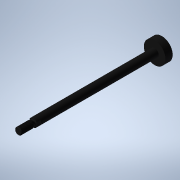
# Autodesk Inventor part: 1463250 DSBC-32-100_(K)
Saved by Autodesk Inventor 2021 (Build 250183000, 183)
## iProperties
Created: 2025-06-06
Part Number: 1463250 DSBC-32-100_(K)
Material: Generic
Catalog Web Link: www.cadenas.de
Description: DSBC_K-Standard cylinder
Vendor: FESTO
Document SubType Name: Modeling
Designer: psAdmin
Manufacturer: FESTO
Mass: 30.5799 g
Surface Area: 101.586 cm^2
Volume: 30.5799 cm^3
Density: 1 g/cm^3
Appearance: PSOLRGB-128-128-128
Category: PARTsolutions
Company: FESTO
Title: 1463250 DSBC-32-100_(K)
Author: Cadenas PARTsolutions
Comments: Standard cylinder
PSOL_IDENT_0: {$CADENAS_DATA/23d-libs/festo/parts/d/dsbc/parts/dsbc_kst.prj},223 {VTYP=3D},{NB=1463250 DSBC-32-100
PSOL_IDENT_1: _(K)},{LINA=1463250 DSBC-32-100_(K)},{NN=DSBC_K},{DATE=30.04.2025 10:56:01},{GEOMDATE=14.10.2015 11:
PSOL_IDENT_2: 10:00},{VERSION=},{LINEID=10},{WBVAR=HUB,VER,FES,KA,KGA,PAR,EG,EK},{WBNUMERIC=HUB,EG,EK}  {NB=146325
PSOL_IDENT_3: 0 DSBC-32-100_(K)},{LINA=1463250 DSBC-32-100_(K)},{KT=DUMMY},{TNR=1463250},{TYP=DSBC},{KDM=32},{HUB=
PSOL_IDENT_4: 100},{HUBMIN=1},{HUBMAX=2800},{VER=-},{VERT=},{FES=-},{FEST=},{KA=-},{KAT=},{KGA=-},{KGAT=},{PAR=-},
PSOL_IDENT_5: {PAR1='-','P2'},{PART=},{EG=0},{EGT=},{A1=35},{EK=0},{EKT=},{A2=0},{A2N=500},{A2P=0},{A=22},{AM=22},
PSOL_IDENT_6: {AF=12},{B=30},{BG=16},{E=45},{EE=G1/8},{EEK=9.728},{G=28.0},{H1=5},{KK=M10x1.25},{KKDM=10.000},{KKP=
PSOL_IDENT_7: 1.250},{L2=18.0},{L3=4.0},{L7=6.5},{L8N=94.000},{L8=194.000},{MM=12},{PL=19.5},{RT=M6},{RTK=6.000},{
PSOL_IDENT_8: TG=32.5},{VA=4},{VD=10.0},{WH=26.0},{ZJN=119.100},{ZJ=219.100},{ZMN=146.100},{ZM=346.100},{SW1=10},{
PSOL_IDENT_9: SW2=16},{SW3=6},{D1=6.4},{KF=M6},{KFK=6.000},{T1=16.0},{T2=2.6},{WL=6.000},{C3=8.200},{D5=1.500},{E2=
PSOL_IDENT_10: 20.000},{F2=0.600},{QH=10.000},{QR=1.000},{W3=45.000},{FDTPIRODACC=4.000},{FDTBDIN439=5.000}
NB: 1463250 DSBC-32-100_(K)
NN: DSBC_K
NT: Standard cylinder
NBSYN: $TNR. $TYP.$VERT.$FEST.-$KDM.-$HUB.$KAT.$KGAT.$PART.$EGT.$EKT._(K)
LINA: 1463250 DSBC-32-100_(K)
CATALOG: Festo
TNR: 1463250
TYP: DSBC
KDM: 32
HUB: 100
HUBMAX: 2800
VER: -
FES: -
KA: -
KGA: -
PAR: -
EG: 0
A1: 35
EK: 0
A2: 0
A2N: 500
A: 22
AM: 22
AF: 12
B: 30
BG: 16
E: 45
EE: G1/8
EEK: 9.728
G: 28
H1: 5
KK: M10x1.25
KKDM: 10
KKP: 1.25
L2: 18
L3: 4
L7: 6.5
L8N: 94
L8: 194
MM: 12
PL: 19.5
RT: M6
RTK: 6
TG: 32.5
VA: 4
VD: 10
WH: 26
ZJN: 119.1
ZJ: 219.1
ZMN: 146.1
ZM: 346.1
SW1: 10
SW2: 16
SW3: 6
D1: 6.4
KF: M6
KFK: 6
T1: 16
T2: 2.6
WL: 6
C3: 8.2
D5: 1.5
E2: 20
F2: 0.6
QH: 10
QR: 1
W3: 45
FDTPIRODACC: 4
FDTBDIN439: 5
SUPPLIER: FESTO
ARTICLENO: 1463250 DSBC-32-100_(K)
BOMINFO: 1463250 DSBC-32-100_(K)
CREATOR: CADENAS GmbH
Autodesk Inventor part; units mm, degrees
ref_plane "YZ Plane" through (0, 0, 0) normal (1, 0, 0) x (0, 1, 0)
ref_plane "XZ Plane" through (0, 0, 0) normal (0, 1, 0) x (-1, 0, 0)
ref_plane "XY Plane" through (0, 0, 0) normal (0, 0, 1) x (1, 0, 0)
sketch "Sketch_1" plane through (0, 0, 0) normal (1, 0, 0) x (0, 1, 0)
  line L0 (0, -166) -> (0, 25.1)
  line L1 (0, 25.1) -> (5.7172, 25.1)
  line L2 (5.7172, 25.1) -> (6, 24.8172)
  line L3 (6, 24.8172) -> (6, -155.3333)
  line L4 (6, -155.3333) -> (16, -155.3333)
  line L5 (16, -155.3333) -> (16, -166)
  line L6 (16, -166) -> (0, -166)
  line L7 (0, -166) -> (0, 25.1)
  constraints: 16 end point
revolve "Revolution1" add sketch "Sketch_1" angle 360 about axis through (0, 0, -166) along (0, 0, -1)
sketch "Sketch_2" plane through (0, 0, 0) normal (0, 1, 0) x (-1, 0, 0)
  line L0 (10, 39.1) -> (-10, 39.1)
  line L1 (-10, 39.1) -> (-10, 19.1)
  line L2 (-10, 19.1) -> (-5, 19.1)
  line L3 (-5, 19.1) -> (-5, 31.1)
  line L4 (-5, 31.1) -> (5, 31.1)
  line L5 (5, 31.1) -> (5, 19.1)
  line L6 (5, 19.1) -> (10, 19.1)
  line L7 (10, 19.1) -> (10, 39.1)
  constraints: 16 end point
extrude "Extrusion1" cut sketch "Sketch_2" along normal mid plane 20
sketch "Sketch_4" plane through (0, 0, 0) normal (1, 0, 0) x (0, 1, 0)
  line L0 (0, 24.5) -> (0, 47.1)
  line L1 (0, 47.1) -> (4.233, 47.1)
  line L2 (4.233, 47.1) -> (5, 46.333)
  line L3 (5, 46.333) -> (5, 29.0727)
  line L4 (5, 29.0727) -> (4.1362, 26.6994)
  arc A0 (4.1362, 26.6994) -> (4.1, 26.4942) centre (4.7, 26.4942) ccw
  line L5 (4.1, 26.4942) -> (4.1, 25.7)
  arc A1 (4.1, 25.7) -> (4.7, 25.1) centre (4.7, 25.7) ccw
  line L6 (4.7, 25.1) -> (4.7, 24.5)
  line L7 (4.7, 24.5) -> (0, 24.5)
  line L8 (0, 24.5) -> (0, 47.1)
  constraints: 18 end point, 4 point on circle, 2 centre point
revolve "Revolution2" add sketch "Sketch_4" angle 360 about axis through (0, 0, 24.5) along (0, 0, -1)
thread "Thread1" size "M10x1.25" class "6g" standard "ISO Metric profile" full length
ref_plane "FDT_PIRODACC_XY" through (0, 0, 34.1) normal (0, 0, 1) x (1, 0, 0)
ref_plane "FDT_PIRODACC_YZ" through (0, 0, 34.1) normal (1, 0, 0) x (0, 1, 0)
ref_plane "FDT_PIRODACC_ZX" through (0, 0, 34.1) normal (0, 1, 0) x (0, 0, 1)
ref_plane "NUT_XY" through (0, 0, 34.1) normal (0, 0, -1) x (1, 0, 0)
ref_plane "NUT_YZ" through (0, 0, 34.1) normal (1, 0, 0) x (0, -1, 0)
ref_plane "NUT_ZX" through (0, 0, 34.1) normal (0, -1, 0) x (0, 0, -1)
ref_plane "P_XY" through (0, 0, -166) normal (0, 0, -1) x (0, 1, 0)
ref_plane "P_YZ" through (0, 0, -166) normal (0, 1, 0) x (1, 0, 0)
ref_plane "P_ZX" through (0, 0, -166) normal (1, 0, 0) x (0, 0, -1)
body "Solid1"
